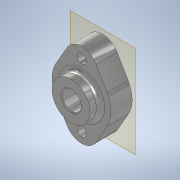
# Autodesk Inventor part: Фланецгайка
Saved by Autodesk Inventor 2021 (Build 250183000, 183)
## iProperties
Created: 2020-12-01
Part Number: Фланецгайка
Material: Сталь, углеродистая
Document SubType Name: Modeling
Designer: Тимоха
Density: 7.85 g/cm^3
Appearance: С умеренной полировкой
Mass: 8696.9 g
Surface Area: 893.705 cm^2
Volume: 1107.89 cm^3
Author: Тимоха
Autodesk Inventor part; units mm, degrees
ref_plane "YZ Plane" through (0, 0, 0) normal (1, 0, 0) x (0, 1, 0)
ref_plane "XZ Plane" through (0, 0, 0) normal (0, 1, 0) x (-1, 0, 0)
ref_plane "XY Plane" through (0, 0, 0) normal (0, 0, 1) x (1, 0, 0)
ref_plane "РабПлоскость1" through (0, 0, 0) normal (0, 0, 1) x (1, 0, 0)
sketch "Эскиз1" plane through (0, 0, 0) normal (0, 0, 1) x (1, 0, 0)
  circle A0 centre (0, 75) radius 8 projected
  circle A1 centre (0, -75) radius 8 projected
  line L0 (34.641, -80) -> (60.6218, -35) projected
  arc A2 (60.6218, -35) -> (60.6218, 35) centre (0, 0) ccw projected
  line L1 (60.6218, 35) -> (34.641, 80) projected
  arc A3 (34.641, 80) -> (-34.641, 80) centre (0, 60) ccw projected
  line L2 (-34.641, 80) -> (-60.6218, 35) projected
  arc A4 (-60.6218, 35) -> (-60.6218, -35) centre (0, 0) ccw projected
  line L3 (-60.6218, -35) -> (-34.641, -80) projected
  arc A5 (-34.641, -80) -> (34.641, -80) centre (0, -60) ccw projected
  circle A6 centre (0, 0) radius 50 projected
  circle A7 centre (0, 75) radius 11
  circle A8 centre (0, -75) radius 11
  point P0 (0, 0)
  dimension "d22" = 22
  dimension "d23" = 22
  constraints: 2 centre point, 2 coincident
  measures "d22" diameter of A7
  measures "d23" diameter of A8
extrude "Выдавливание1" add sketch "Эскиз1" along normal blind 50 contours A5 L3 A4 L2 A3 L1 A2 L0 | A6
sketch "Эскиз2" plane through (0, 0, 0) normal (0, 0, -1) x (-1, 0, 0)
  circle A0 centre (0, 0) radius 50
  dimension "d2" = 100
  constraints: 1 centre point, 1 coincident
  measures "d2" diameter of A0
extrude "Выдавливание2" add sketch "Эскиз2" along normal blind 15
sketch "Эскиз3" plane through (0, 0, 50) normal (0, 0, 1) x (1, 0, 0)
  circle A0 centre (0, 0) radius 45
  dimension "d5" = 90
  constraints: 1 centre point, 1 coincident
  measures "d5" diameter of A0
extrude "Выдавливание3" add sketch "Эскиз3" along normal blind 25
fillet "Сопряжение1" radius 10 1 edges at (-45, 0, 50)
sketch "Эскиз4" plane through (0, 0, 75) normal (0, 0, 1) x (1, 0, 0)
  circle A0 centre (0, 0) radius 55 projected
  circle A1 centre (0, 0) radius 22.5
  dimension "d9" = 45
  constraints: 1 centre point, 1 coincident
  measures "d9" diameter of A1
extrude "Выдавливание4" cut sketch "Эскиз4" against normal through all contours A1
chamfer "Фаска1" distance 2 angle 45 3 edges at (-22.5, 0, 75) (50, 0, -15) (-22.5, 0, -15)
sketch "Эскиз5" plane through (0, 0, 0) normal (1, 0, 0) x (0, 1, 0)
  line L0 (-24.5, -15) -> (24.5, -15) projected
  line L1 (48, -15) -> (-48, -15) projected
  line L2 (22.5, 73) -> (22.5, -13) projected
  line L3 (22.5, -15) -> (22.5, -8)
  line L4 (22.5, -8) -> (27.5, -8)
  line L5 (27.5, -8) -> (29.3756, -15)
  line L6 (0, -32.6) -> (0, 90.6) projected
  point P0 (0, 0)
  dimension "d15" = 7
  dimension "d16" = 5
  dimension "d17" = 105
  constraints: 6 end point, 3 point on line, 1 perpendicular
  measures "d15" distance of L3.start L3.end
  measures "d16" distance of L3.end L4.end
  measures "d17" angle of L4 L5
revolve "Вращение1" cut sketch "Эскиз5" angle 360 about axis through (0, 0, -10) along (0, 0, 1)
chamfer "Фаска2" distance 2 angle 45 1 edges at (-22.5, 0, -8)
